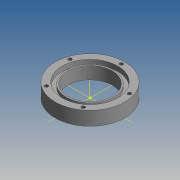
# Autodesk Inventor part: P029_BasEcranProtecCam
Saved by Autodesk Inventor 2021.3 (Build 253353000, 353)
## iProperties
Created: 2021-11-19
Part Number: P029_BasEcranProtecCam
Material: Générique
Document SubType Name: Modeling
Designer: gabri
Density: 1 g/cm^3
Appearance: Par défaut
Author: gabri
Autodesk Inventor part; units mm, degrees
ref_plane "YZ Plane" through (0, 0, 0) normal (1, 0, 0) x (0, 1, 0)
ref_plane "XZ Plane" through (0, 0, 0) normal (0, 1, 0) x (-1, 0, 0)
ref_plane "XY Plane" through (0, 0, 0) normal (0, 0, 1) x (1, 0, 0)
sketch "Sketch2" plane through (0, 0, 0) normal (0, 0, 1) x (1, 0, 0)
  circle A0 centre (0, 0) radius 25
  circle A1 centre (0, 0) radius 16
  dimension "d0" = 50
  dimension "d1" = 32
  constraints: 2 centre point, 2 coincident
  measures "d0" diameter of A0
  measures "d1" diameter of A1
extrude "Extrusion1" add sketch "Sketch2" along normal blind 10
sketch "Sketch3" plane through (0, 0, 10) normal (0, 0, 1) x (1, 0, 0)
  circle A0 centre (0, 0) radius 25 construction
  circle A1 centre (0, 0) radius 16 construction
  circle A2 centre (0, 0) radius 16
  circle A3 centre (0, 0) radius 20
  dimension "d4" = 4
  constraints: 2 centre point, 2 coincident, 1 concentric
  measures "d4" radial gap between concentric circles of A1 A3
extrude "Extrusion2" cut sketch "Sketch3" against normal blind 1
sketch "Sketch4" plane through (0, 0, 9) normal (0, 0, 1) x (1, 0, 0)
  circle A0 centre (0, 0) radius 20 construction
  circle A1 centre (0, 0) radius 16 construction
  circle A2 centre (0, 0) radius 20
  circle A3 centre (0, 0) radius 17
  dimension "d7" = 1
  dimension "d8" = 40
  dimension "d9" = 34
  constraints: 2 centre point, 1 coincident, 1 concentric
  measures "d7" radial gap between concentric circles of A1 A3
  measures "d8" diameter of A2
  measures "d9" diameter of A3
extrude "Extrusion3" cut sketch "Sketch4" against normal blind 2.5
sketch "Sketch5" plane through (0, 0, 10) normal (0, 0, 1) x (1, 0, 0)
  line L0 (0, 35) -> (0, -35) construction
  circle A0 centre (0, 0) radius 20 construction
  point P0 (0, 22.5)
  point P1 (-21.3988, 6.9529)
  point P2 (-13.2252, -18.2029)
  point P3 (13.2252, -18.2029)
  point P4 (21.3988, 6.9529)
  dimension "d12" = 22.5
  dimension "d15" = 360
  constraints: 1 point on line, 6 other
  measures "d12" distance of A0.centre point (0, 22.5)
hole "Hole1" at (-21.3988, 6.9529, 10) at (0, 22.5, 10) at (21.3988, 6.9529, 10) at (13.2252, -18.2029, 10) at (-13.2252, -18.2029, 10) direction (0, 0, -1) diameter 2.459 depth 8.8 tip angle 118 thread size "M3x0.5" class "6H" standard "ISO Metric profile"
body "Solid1"
